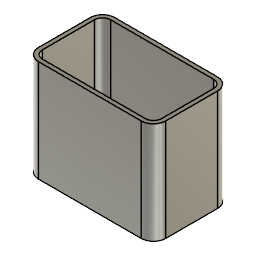
▢-125×75×4.0 (Autodesk Fusion 360 design; units mm, degrees)
Autodesk Fusion 360 part; units mm, degrees
sketch "スケッチ1" plane through (0, 0, 0) normal (0, 0, 1) x (1, 0, 0)
  line L0 (347.8927, 333.8164) -> (448.8927, 333.8164)
  line L1 (347.8927, 337.8164) -> (448.8927, 337.8164)
  line L2 (448.8927, 408.8164) -> (347.8927, 408.8164)
  line L3 (448.8927, 404.8164) -> (347.8927, 404.8164)
  line L4 (335.8927, 396.8164) -> (335.8927, 345.8164)
  line L5 (339.8927, 396.8164) -> (339.8927, 345.8164)
  arc A0 (335.8927, 345.8164) -> (347.8927, 333.8164) centre (347.8927, 345.8164) ccw
  arc A1 (339.8927, 345.8164) -> (347.8927, 337.8164) centre (347.8927, 345.8164) ccw
  arc A2 (347.8927, 408.8164) -> (335.8927, 396.8164) centre (347.8927, 396.8164) ccw
  arc A3 (347.8927, 404.8164) -> (339.8927, 396.8164) centre (347.8927, 396.8164) ccw
  line L6 (460.8927, 345.8164) -> (460.8927, 396.8164)
  line L7 (456.8927, 345.8164) -> (456.8927, 396.8164)
  arc A4 (448.8927, 333.8164) -> (460.8927, 345.8164) centre (448.8927, 345.8164) ccw
  arc A5 (448.8927, 337.8164) -> (456.8927, 345.8164) centre (448.8927, 345.8164) ccw
  arc A6 (460.8927, 396.8164) -> (448.8927, 408.8164) centre (448.8927, 396.8164) ccw
  arc A7 (456.8927, 396.8164) -> (448.8927, 404.8164) centre (448.8927, 396.8164) ccw
  point P0 (398.3927, 371.3164)
extrude "押し出し1" add sketch "スケッチ1" along normal blind 100
